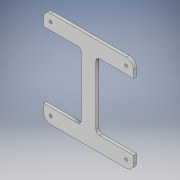
# Autodesk Inventor part: HeadBasePlate
Saved by Autodesk Inventor 2019 (Build 230136000, 136)
## iProperties
Created: 2019-06-11
Part Number: HeadBasePlate
Material: Generic
Document SubType Name: Modeling
Designer: Cole
Density: 1 g/cm^3
Appearance: Default
Author: Cole
Autodesk Inventor part; units mm, degrees
ref_plane "YZ Plane" through (0, 0, 0) normal (1, 0, 0) x (0, 1, 0)
ref_plane "XZ Plane" through (0, 0, 0) normal (0, 1, 0) x (-1, 0, 0)
ref_plane "XY Plane" through (0, 0, 0) normal (0, 0, 1) x (1, 0, 0)
sketch "Sketch1" plane through (0, 0, 0) normal (0, 0, 1) x (1, 0, 0)
  line L0 (32.3895, 41.275) -> (-32.3895, 41.275) projected
  line L1 (38.7395, -34.925) -> (38.7395, 34.925) projected
  circle A0 centre (-32.3895, 34.925) radius 1.25 projected
  circle A1 centre (32.3895, 34.925) radius 1.25 projected
  circle A2 centre (32.3895, -34.925) radius 1.25 projected
  circle A3 centre (-32.3895, -34.925) radius 1.25 projected
  arc A4 (38.7395, 34.925) -> (32.3895, 41.275) centre (32.3895, 34.925) ccw
  line L2 (-32.3895, -41.275) -> (32.3895, -41.275) projected
  line L3 (-38.7395, 34.925) -> (-38.7395, -34.925) projected
  arc A5 (-32.3895, 41.275) -> (-38.7395, 34.925) centre (-32.3895, 34.925) ccw projected
  arc A6 (-38.7395, -34.925) -> (-32.3895, -41.275) centre (-32.3895, -34.925) ccw projected
  arc A7 (32.3895, -41.275) -> (38.7395, -34.925) centre (32.3895, -34.925) ccw projected
  point P0 (0, 0)
  constraints: 2 point on circle, 2 tangent, 1 centre point
extrude "Extrusion1" add sketch "Sketch1" along normal blind 2.54
sketch "Sketch2" plane through (0, 0, 2.54) normal (0, 0, 1) x (1, 0, 0)
  line L0 (-38.7395, 28.575) -> (-9.525, 28.575)
  line L1 (-6.35, 25.4) -> (-6.35, -25.4)
  line L2 (-9.525, -28.575) -> (-38.7395, -28.575)
  line L3 (-38.7395, -28.575) -> (-38.7395, 28.575)
  line L4 (38.7395, 28.575) -> (9.525, 28.575)
  line L5 (6.35, 25.4) -> (6.35, -25.4)
  line L6 (9.525, -28.575) -> (38.7395, -28.575)
  line L7 (38.7395, -28.575) -> (38.7395, 28.575)
  line L8 (-38.7395, 34.925) -> (-38.7395, -34.925) projected
  line L9 (38.7395, -34.925) -> (38.7395, 34.925) projected
  circle A0 centre (32.3895, 34.925) radius 1.25 projected
  line L10 (32.3895, 41.275) -> (-32.3895, 41.275) projected
  circle A1 centre (32.3895, -34.925) radius 1.25 projected
  arc A2 (-6.35, 25.4) -> (-9.525, 28.575) centre (-9.525, 25.4) ccw
  arc A3 (-9.525, -28.575) -> (-6.35, -25.4) centre (-9.525, -25.4) ccw
  arc A4 (6.35, -25.4) -> (9.525, -28.575) centre (9.525, -25.4) ccw
  arc A5 (9.525, 28.575) -> (6.35, 25.4) centre (9.525, 25.4) ccw
  point P0 (0, 0)
  point P1 (6.35, -28.575)
  dimension "d2" = 6.35
  dimension "d3" = 6.35
  dimension "d5" = 6.35
  dimension "d6" = 6.35
  dimension "d7" = 6.35
  dimension "d8" = 3.175
  constraints: 16 end point, 8 point on circle, 8 tangent, 6 point on line, 4 centre point, 4 parallel, 3 equal radius, 2 horizontal, 2 perpendicular
  measures "d2" distance from line of A0.centre L4
  measures "d3" distance from line of A0.centre L10
  measures "d5" distance from line of L6 A1.centre
  measures "d6" distance from line of L5 point (0, 0)
  measures "d7" distance from line of L1 point (0, 0)
  measures "d8" radius of A2
extrude "Extrusion2" cut sketch "Sketch2" against normal blind 2.54 contours L0 A2 L1 A3 L2 L3 | L7 L6 A4 L5 A5 L4
equation "\"d2\" = d3"
equation "\"d5\" = d2"
equation "\"d6\" = d5"
equation "\"d7\" = d6"
body "Solid1"
